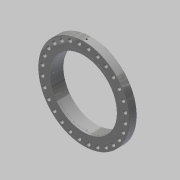
# Autodesk Inventor part: A1-19037-200-04 30in CL300 RF flange - custom
Saved by Autodesk Inventor 2017.3 (Build 213257000, 257)
## iProperties
Created: 2011-05-31
Part Number: A1-19037-200-04 30in CL300 RF flange - custom
Document SubType Name: Modeling
Designer: Graeme_Van_Dongen
Density: 7.85 g/cm^3
Description: 30" CLASS 300 B16.47 Ser.A RFSO FLANGE, A105N, Ø31 1/4" BORE
Material: Steel
Mass: 322596 g
Surface Area: 19889.5 cm^2
Volume: 41095.1 cm^3
Appearance: Steel
Project: A1-19037--CNUL Albian CST laterals
Constructed By: Graeme_Van_Dongen
Project Name: CST laterals
Author: Graeme_Van_Dongen
Autodesk Inventor part; units mm, degrees
ref_plane "YZ Plane" through (0, 0, 0) normal (1, 0, 0) x (0, 1, 0)
ref_plane "XY Plane" through (0, 0, 0) normal (0, 0, 1) x (1, 0, 0)
sketch "Sketch1" plane through (0, 0, 0) normal (0, 0, 1) x (1, 0, 0)
  circle A0 centre (0, 0) radius 546.1
  circle A1 centre (0, 0) radius 396.875
  dimension "d0" = 1092.2
  dimension "d1" = 793.75
  constraints: 2 centre point, 2 coincident
  measures "d0" diameter of A0
  measures "d1" diameter of A1
extrude "Extrusion1" add sketch "Sketch1" along normal blind 90.4875
sketch "Sketch2" plane through (0, 0, 90.4875) normal (0, 0, 1) x (1, 0, 0)
  circle A0 centre (0, 0) radius 396.875 projected
  circle A1 centre (0, 0) radius 546.1 projected
  circle A2 centre (0, 0) radius 428.625
  dimension "d4" = 857.25
  constraints: 1 centre point, 1 coincident
  measures "d4" diameter of A2
extrude "Extrusion2" add sketch "Sketch2" along normal blind 1.5875 contours A2
sketch "Sketch3" plane through (0, 0, 0) normal (0, 0, -1) x (-1, 0, 0)
  circle A0 centre (0, 0) radius 396.875 projected
  circle A1 centre (0, 0) radius 546.1 projected
  circle A2 centre (0, 0) radius 441.325
  dimension "d7" = 882.65
  constraints: 1 centre point, 1 coincident
  measures "d7" diameter of A2
extrude "Extrusion3" add sketch "Sketch3" along normal blind 61.9125 contours A2
sketch "Sketch4" plane through (0, 0, 92.075) normal (0, 0, 1) x (1, 0, 0)
  line L0 (0, 0) -> (55.8115, 495.3407) construction
  line L1 (0, -764.54) -> (0, 764.54) construction
  dimension "d13" = 498.475
  dimension "d99" = 6.429
  constraints: 2 end point
  measures "d13" distance of L0.start L0.end
  measures "d99" angle of L0 L1
hole "Hole1" at (55.8115, 495.3407, 92.075) direction (0, 0, -1) diameter 47.625 end through all
chamfer "Chamfer3" distance 0.7937 angle 45 2 edges at (55.8115, 519.1532, 0) (55.8115, 519.1532, 90.4875)
pattern_circular "Circular Pattern1" count 28 over 360 about axis through (0, 0, -10) along (0, 0, -1) of "Hole1", "Chamfer3"
chamfer "Chamfer2" distance 1.5875 angle 45 2 edges at (-546.1, 0, 0) (-546.1, 0, 90.4875)
fillet "Fillet2" radius 11.1125 1 edges at (441.325, 0, 0)
chamfer "Chamfer4" distance 1.5875 angle 45 1 edges at (441.325, 0, -61.9125)
sketch "Sketch6" plane through (0, 0, 0) normal (1, 0, 0) x (0, 1, 0)
  line L0 (441.325, -11.1125) -> (441.325, -60.325) construction
  line L1 (439.7375, -61.9125) -> (-439.7375, -61.9125) construction
  line L2 (431.8, -42.1631) -> (414.3375, -55.5625)
  line L3 (411.1625, -61.9125) -> (441.325, -61.9125)
  line L4 (0, -85.725) -> (0, 114.3) projected
  line L5 (411.1625, -61.9125) -> (411.1625, -55.5625)
  line L6 (396.875, -61.9125) -> (396.875, 92.075) construction
  line L7 (411.1625, -55.5625) -> (414.3375, -55.5625)
  line L8 (396.875, 92.075) -> (400.05, 92.075)
  line L9 (400.05, 92.075) -> (400.05, 66.675)
  line L10 (400.05, 66.675) -> (396.875, 66.675)
  line L11 (396.875, 66.675) -> (396.875, 92.075)
  line L12 (431.8, -42.1631) -> (431.8, -36.5125)
  line L13 (441.325, -24.2158) -> (441.325, -61.9125)
  arc A0 (441.325, -24.2158) -> (431.8, -36.5125) centre (444.5, -36.5125) ccw
  point P0 (0, 0)
  dimension "d45" = 37.5
  dimension "d59" = 6.35
  dimension "d69" = 17.4625
  dimension "d70" = 3.175
  dimension "d71" = 25.4
  dimension "d72" = 400.05
  dimension "d96" = 431.8
  dimension "d97" = 12.7
  dimension "d98" = 25.4
  constraints: 21 end point, 3 collinear, 3 parallel, 2 horizontal, 2 point on circle, 2 point on line, 1 centre point, 1 perpendicular, 1 tangent, 1 vertical
  measures "d45" angle of L3 L2
  measures "d59" distance of L3.start L5.end
  measures "d69" horizontal distance of L2.start L2.end
  measures "d70" distance of L5.end L2.end
  measures "d71" distance from line of L6.end L10
  measures "d72" distance from line of point (0, 0) L9
  measures "d96" distance between parallel lines of L4 L12
  measures "d97" radius of A0
  measures "d98" distance from line of A0.centre L3
revolve "Revolution1" cut sketch "Sketch6" angle 360 about axis through (0, 0, -10) along (0, 0, 1)
fillet "Fillet5" radius 0.7937 1 edges at (0, -400.05, 66.675)
chamfer "Chamfer7" distance 0.7937 angle 45 1 edges at (-396.875, 0, 66.675)
ref_plane "Work Plane1" through (0, 546.1, 0) normal (0, 1, 0) x (-1, 0, 0)
sketch "Sketch11" plane through (0, 546.1, 0) normal (0, 1, 0) x (-1, 0, 0)
  line L0 (-399.2563, 66.675) -> (399.2563, 66.675) construction
  line L1 (397.6687, 66.675) -> (-397.6687, 66.675) construction
  point P0 (0, 0)
  point P1 (0, 53.975)
  dimension "d101" = 12.7
  constraints: 1 vertical alignment
  measures "d101" distance from line of L0 point (0, 53.975)
hole "Hole4" at (0, 546.1, 53.975) direction (0, -1, 0) diameter 17.4752 depth 27.94 tip angle 118 thread size "1/2" designation "1/2 - 14 NPT" standard "NPT"
hole "Hole5" at (0, 546.1, 53.975) direction (0, -1, 0) diameter 10.5918 depth 44.45 tip angle 118 thread size "1/2-13 UNC" class "2B" standard "ANSI Unified Screw Threads"
hole "Hole6" at (0, 546.1, 53.975) direction (0, -1, 0) diameter 10.3188 depth 152.4 tip angle 118
pattern_circular "Circular Pattern3" count 4 over 360 about axis through (0, 0, -10) along (0, 0, 1) of "Hole4", "Hole5", "Hole6"
equation "\"d0\" = OD"
equation "\"d1\" = Bore"
equation "\"d2\" = Thickness"
equation "\"d4\" = RFDia"
equation "\"d5\" = RFDepth"
equation "\"d7\" = NeckDia"
equation "\"d8\" = NeckLength"
equation "\"d13\" = 0.5 * BCD"
equation "\"d15\" = HoleDia"
equation "\"d30\" = HoleChamfer"
equation "\"d25\" = RimChamfer"
equation "\"d29\" = NeckFillet"
equation "\"d33\" = NeckChamfer"
equation "\"d72\" = 0.5 * Bore + Lockstep"
equation "\"d96\" = 0.5 * Casing"
equation "\"OD\" = 1092.2"
equation "\"Bore\" = 793.75"
equation "\"Thickness\" = 90.4875"
equation "\"RFDia\" = 857.25"
equation "\"RFDepth\" = 1.5875"
equation "\"HoleDia\" = 47.625"
equation "\"BCD\" = 996.95"
equation "\"NeckDia\" = 882.65"
equation "\"NeckLength\" = 61.9125"
equation "\"HoleChamfer\" = 0.79375"
equation "\"RimChamfer\" = 1.5875"
equation "\"NeckChamfer\" = 1.5875"
equation "\"NeckFillet\" = 11.1125"
equation "\"Lock\" = 25.4"
equation "\"Lockstep\" = 3.175"
equation "\"Size\" = 762"
equation "\"Wall\" = 19.05"
equation "\"Casing\" = 863.6"
body "Solid1"
